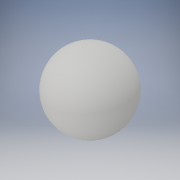
# Autodesk Inventor part: DraftOfBoulder
Saved by Autodesk Inventor 2017 (Build 210142000, 142)
## iProperties
Created: 2016-01-12
Part Number: DraftOfBoulder
Material: Generic
Document SubType Name: Modeling
Designer: steele
Density: 1 g/cm^3
Appearance: Default
Mass: 8580.25 g
Surface Area: 2026.83 cm^2
Volume: 8580.25 cm^3
Author: steele
Autodesk Inventor part; units mm, degrees
ref_plane "YZ Plane" through (0, 0, 0) normal (1, 0, 0) x (0, 1, 0)
ref_plane "XZ Plane" through (0, 0, 0) normal (0, 1, 0) x (-1, 0, 0)
sketch "Sketch1" plane through (0, 0, 0) normal (0, 0, 1) x (1, 0, 0)
  arc A0 (0, -127) -> (0, 127) centre (0, 0) ccw
  line L0 (0, 127) -> (0, -127)
  dimension "d0" = 254
  constraints: 2 end point, 2 point on circle, 1 centre point, 1 coincident, 1 vertical
  measures "d0" diameter of A0
revolve "Revolution1" add sketch "Sketch1" angle 360 about axis through (0, 127, 0) along (0, -1, 0)
ref_plane "Work Plane2" through (0, 0, -127) normal (0, 0, 1) x (1, 0, 0)
ref_plane "Work Plane1" through (0, 0, 127) normal (0, 0, 1) x (1, 0, 0)
equation "\"d0\" = boulderDiam"
equation "\"boulderDiam\" = 254"
body "Solid1"
